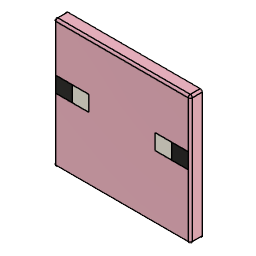
front_face_plate (Autodesk Fusion 360 design; units mm, degrees)
part number: 2025-10-11-08-44-41-819
Autodesk Fusion 360 part; units mm, degrees
note: some values were not read from the file. Set by a fixed rule: which sketch regions a step uses.
sketch "Front Face Plate" plane through (0, 0, 0) normal (0, 1, 0) x (1, 0, 0)
  line L0 (0, 0) -> (136, 0)
  line L1 (136, 0) -> (136, -128)
  line L2 (136, -128) -> (0, -128)
  line L3 (0, -128) -> (0, 0)
  dimension "d5" = 136
  dimension "d6" = 128
  constraint horizontal L0
  constraint vertical L1
  constraint horizontal L2
  constraint vertical L3
  constraint coincident L0.start L3.end
  measures "d5" distance of L0.start L0.end
  measures "d6" distance of L0.start L2.end
extrude "Extrude1" add sketch "Front Face Plate" along normal blind 12 makes body 1
sketch "Eyes" plane through (0, 0, 0) normal (0, -1, 0) x (1, 0, 0)
  line L0 (136, 128) -> (0, 128)
  line L1 (0, 128) -> (0, 0)
  line L2 (0, 0) -> (136, 0)
  line L3 (136, 0) -> (136, 128)
  line L4 (2, 79.5) -> (18.5, 79.5)
  line L5 (18.5, 79.5) -> (18.5, 64)
  line L6 (18.5, 64) -> (2, 64)
  line L7 (2, 64) -> (2, 79.5)
  line L8 (18.5, 79.5) -> (35, 79.5)
  line L9 (35, 79.5) -> (35, 64)
  line L10 (35, 64) -> (18.5, 64)
  line L11 (18.5, 64) -> (18.5, 79.5)
  line L12 (101, 79.5) -> (117.5, 79.5)
  line L13 (117.5, 79.5) -> (117.5, 64)
  line L14 (117.5, 64) -> (101, 64)
  line L15 (101, 64) -> (101, 79.5)
  line L16 (117.5, 79.5) -> (134, 79.5)
  line L17 (134, 79.5) -> (134, 64)
  line L18 (134, 64) -> (117.5, 64)
  line L19 (117.5, 64) -> (117.5, 79.5)
  dimension "d10" = 16.5
  dimension "d11" = 16.5
  dimension "d12" = 16.5
  dimension "d13" = 16.5
  dimension "d14" = 15.5
  dimension "d15" = 15.5
  dimension "d16" = 48.5
  dimension "d17" = 48.5
  dimension "d23" = 2
  dimension "d24" = 2
  constraint horizontal L4
  constraint vertical L5
  constraint horizontal L6
  constraint vertical L7
  constraint horizontal L8
  constraint vertical L9
  constraint horizontal L10
  constraint vertical L11
  constraint horizontal L12
  constraint vertical L13
  constraint horizontal L14
  constraint vertical L15
  constraint horizontal L16
  constraint vertical L17
  constraint horizontal L18
  constraint vertical L19
  constraint collinear L6 L10
  constraint collinear L14 L18
  measures "d10" distance of L4.start L4.end
  measures "d11" distance of L4.end L8.end
  measures "d12" distance of L12.start L12.end
  measures "d13" distance of L12.end L16.end
  measures "d14" distance of L8 L10
  measures "d15" distance of L12.start L14.end
  measures "d16" distance of L0 L4
  measures "d17" distance of L0 L16
  measures "d23" distance of L1 L7
  measures "d24" distance of L3 L17
extrude "Extrude2" add sketch "Eyes" along normal blind 0.01 separate body contours L4 L5 L6 L7 L11 | L13 L16 L17 L18 L19 makes body 2 at (7.5, 0, 74.3333) makes body 3 at (128.5, 0, 69.1667)
extrude "Extrude3" add sketch "Eyes" along normal blind 0.01 separate body contours L5 L8 L9 L10 L11 | L12 L13 L14 L15 L19 makes body 4 at (24, 0, 74.3333) makes body 5 at (106.5, 0, 69.1667)
fillet "Fillet1" radius 2 8 edges at (136, 6, 128) (0, 6, 128) (136, 6, 0) (0, 6, 0) (68, 0, 0) (0, 0, 64) (68, 0, 128) (136, 0, 64) on bodies 1
equation "block_size = 16 mm" comment "The size of the blocks used for the dimensions of the Minecraft Pig."
equation "pine_thickness = 12 mm" comment "The thickness of the pine boards used for the Minecraft Pig's body."
equation "front_face_plate_height = 8 * block_size" comment "The height of the Front Face Plate that makes up the Minecraft Pig's face."
equation "front_face_plate_width = 10 * block_size - 2 * pine_thickness" comment "The width of the Front Face Plate that makes up the Minecraft Pig's face."
equation "d5 = front_face_plate_width"
equation "d6 = front_face_plate_height"
equation "d7 = pine_thickness"
equation "face_block_width = ( front_face_plate_width - 2 * fillet_radius ) / 8" comment "The width of the blocks used for the Minecraft Pig's eyes."
equation "d10 = face_block_width"
equation "d11 = face_block_width"
equation "d12 = face_block_width"
equation "d13 = face_block_width"
equation "d14 = face_block_height"
equation "d15 = face_block_height"
equation "d16 = ( 3 * face_block_height ) + fillet_radius"
equation "d17 = ( 3 * face_block_height ) + fillet_radius"
equation "fillet_radius = 2 mm" comment "The radius of the fillets applied to the Front Face Plate."
equation "d23 = fillet_radius"
equation "d24 = fillet_radius"
equation "d26 = fillet_radius"
equation "face_block_height = ( front_face_plate_height - 2 * fillet_radius ) / 8" comment "The height of the blocks used for the Minecraft Pig's eyes."
named bodies: "Front Face Plate", "Right Eye Pupil", "Left Eye Pupil", "Right Eye White", "Left Eye White"
